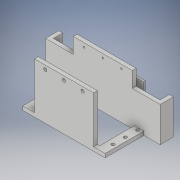
# Autodesk Inventor part: Frame
Saved by Autodesk Inventor 2019 (Build 230136000, 136)
## iProperties
Created: 2018-11-05
Part Number: Frame
Material: 일반
Document SubType Name: Modeling
Designer: otm09
Density: 1 g/cm^3
Appearance: 기본값
Author: otm09
Autodesk Inventor part; units mm, degrees
ref_plane "YZ Plane" through (0, 0, 0) normal (1, 0, 0) x (0, 1, 0)
ref_plane "XZ Plane" through (0, 0, 0) normal (0, 1, 0) x (-1, 0, 0)
ref_plane "XY Plane" through (0, 0, 0) normal (0, 0, 1) x (1, 0, 0)
sketch "스케치1" plane through (0, 0, 0) normal (0, 1, 0) x (-1, 0, 0)
  line L0 (0, 0) -> (106, 0)
  line L1 (106, 0) -> (106, -67)
  line L2 (106, -67) -> (0, -67)
  line L3 (0, -67) -> (0, 0)
  circle A0 centre (5, -15) radius 1.1
  circle A1 centre (5, -31) radius 1.1
  circle A2 centre (5, -47) radius 1.1
  circle A3 centre (101, -15) radius 1.1
  circle A4 centre (101, -31) radius 1.1
  circle A5 centre (101, -47) radius 1.1
  dimension "d1" = 2.2
  dimension "d4" = 16
  dimension "d7" = 96
  dimension "d10" = 5
  dimension "d11" = 15
  dimension "d12" = 5
  dimension "d13" = 20
  constraints: 8 end point, 6 centre point, 2 horizontal, 2 parallel, 1 perpendicular, 1 vertical, 10 other
  measures "d1" diameter of A0
  measures "d4" distance of A0.centre A1.centre
  measures "d7" distance of A0.centre A3.centre
  measures "d10" distance from line of L3 A0.centre
  measures "d11" distance from line of L0 A0.centre
  measures "d12" distance from line of L1 A3.centre
  measures "d13" distance from line of A2.centre L2
extrude "돌출1" add sketch "스케치1" along normal blind 5
sketch "스케치2" plane through (0, 5, 0) normal (0, 1, 0) x (1, 0, 0)
  circle A0 centre (-5, 15) radius 1.1 projected
  circle A1 centre (-5, 15) radius 2.1
  circle A2 centre (-5, 31) radius 1.1 projected
  circle A3 centre (-5, 31) radius 2.1
  circle A4 centre (-5, 47) radius 1.1 projected
  circle A5 centre (-5, 47) radius 2.1
  circle A6 centre (-101, 47) radius 1.1 projected
  circle A7 centre (-101, 47) radius 2.1
  circle A8 centre (-101, 31) radius 1.1 projected
  circle A9 centre (-101, 31) radius 2.1
  circle A10 centre (-101, 15) radius 1.1 projected
  circle A11 centre (-101, 15) radius 2.1
  point P0 (0, 0)
  dimension "d16" = 4.2
  dimension "d17" = 4.2
  dimension "d18" = 4.2
  dimension "d19" = 4.2
  dimension "d20" = 4.2
  dimension "d21" = 4.2
  constraints: 6 centre point, 6 coincident
  measures "d16" diameter of A1
  measures "d17" diameter of A3
  measures "d18" diameter of A5
  measures "d19" diameter of A7
  measures "d20" diameter of A9
  measures "d21" diameter of A11
extrude "돌출2" cut sketch "스케치2" against normal blind 3
sketch "스케치3" plane through (0, 5, 0) normal (0, 1, 0) x (1, 0, 0)
  line L0 (-106, 67) -> (0, 67) projected
  line L1 (-106, 0) -> (0, 0) projected
  line L2 (-91, 67) -> (-15, 67)
  line L3 (-15, 67) -> (-15, 0)
  line L4 (-15, 0) -> (-91, 0)
  line L5 (-91, 0) -> (-91, 67)
  line L6 (0, 0) -> (0, 67) projected
  line L7 (-106, 67) -> (-106, 0) projected
  line L8 (-91, 0) -> (-15, 0)
  line L9 (-15, 0) -> (-15, 5)
  line L10 (-15, 5) -> (-91, 5)
  line L11 (-91, 5) -> (-91, 0)
  line L12 (-91, 55) -> (-15, 55)
  line L13 (-15, 55) -> (-15, 50)
  line L14 (-15, 50) -> (-91, 50)
  line L15 (-91, 50) -> (-91, 55)
  dimension "d24" = 15
  dimension "d25" = 15
  dimension "d26" = 5
  dimension "d27" = 5
  dimension "d30" = 45
  constraints: 24 end point, 6 parallel, 6 point on line, 3 horizontal, 3 perpendicular, 1 collinear
  measures "d24" distance between parallel lines of L6 L3
  measures "d25" distance between parallel lines of L7 L5
  measures "d26" distance of L9.end L8.end
  measures "d27" distance of L12.end L13.end
  measures "d30" distance between parallel lines of L10 L14
extrude "돌출3" add sketch "스케치3" along normal blind 60 contours L12 L3 L14 L5 | L5 L10 L3 L1
sketch "스케치4" plane through (-106, 0, 0) normal (0, 0, 1) x (1, 0, 0)
  circle A0 centre (53, 60) radius 1.1
  circle A1 centre (77, 60) radius 1.1
  circle A2 centre (29, 60) radius 1.1
  line L0 (91, 5) -> (91, 65) projected
  line L1 (15, 65) -> (91, 65) projected
  point P0 (106, 0)
  dimension "d33" = 2.2
  dimension "d34" = 2.2
  dimension "d35" = 2.2
  dimension "d36" = 24
  dimension "d37" = 24
  dimension "d38" = 38
  dimension "d39" = 5
  dimension "d40" = 5
  dimension "d41" = 5
  constraints: 3 centre point
  measures "d33" diameter of A0
  measures "d34" diameter of A1
  measures "d35" diameter of A2
  measures "d36" distance of A2.centre A0.centre
  measures "d37" distance of A1.centre A0.centre
  measures "d38" distance from line of A0.centre L0
  measures "d39" distance from line of A0.centre L1
  measures "d40" distance from line of A1.centre L1
  measures "d41" distance from line of A2.centre L1
extrude "돌출4" cut sketch "스케치4" against normal blind 55
sketch "스케치5" plane through (-106, 0, 0) normal (0, 0, 1) x (1, 0, 0)
  circle A0 centre (29, 60) radius 1.1 projected
  circle A1 centre (29, 60) radius 2.1
  circle A2 centre (53, 60) radius 1.1 projected
  circle A3 centre (53, 60) radius 2.1
  circle A4 centre (77, 60) radius 1.1 projected
  circle A5 centre (77, 60) radius 2.1
  point P0 (106, 0)
  dimension "d44" = 4.2
  dimension "d45" = 4.2
  dimension "d46" = 4.2
  constraints: 3 centre point, 3 coincident
  measures "d44" diameter of A1
  measures "d45" diameter of A3
  measures "d46" diameter of A5
sketch "스케치6" plane through (-15, 5, -55) normal (0, 0, -1) x (-1, 0, 0)
  circle A0 centre (14, 55) radius 1.1 projected
  circle A1 centre (14, 55) radius 2.1
  circle A2 centre (38, 55) radius 1.1 projected
  circle A3 centre (38, 55) radius 2.1
  circle A4 centre (62, 55) radius 1.1 projected
  circle A5 centre (62, 55) radius 2.1
  point P0 (-15, -5)
  dimension "d47" = 4.2
  dimension "d48" = 4.2
  dimension "d49" = 4.2
  constraints: 3 centre point, 3 coincident
  measures "d47" diameter of A1
  measures "d48" diameter of A3
  measures "d49" diameter of A5
extrude "돌출5" cut sketch "스케치6" against normal blind 3
extrude "돌출6" cut sketch "스케치5" against normal blind 3
sketch "스케치7" plane through (0, 5, 0) normal (0, 1, 0) x (1, 0, 0)
  line L0 (-91, 67) -> (-15, 67)
  line L1 (-15, 67) -> (-15, 64.3)
  line L2 (-15, 64.3) -> (-91, 64.3)
  line L3 (-91, 64.3) -> (-91, 67)
  line L4 (-91, 55) -> (-91, 50) projected
  line L5 (-15, 50) -> (-15, 55) projected
  line L6 (-15, 55) -> (-91, 55) projected
  line L7 (-126.75, 50) -> (-121.75, 50)
  line L8 (-121.75, 50) -> (-121.75, 67)
  line L9 (-121.75, 67) -> (-126.75, 67)
  line L10 (-126.75, 67) -> (-126.75, 50)
  line L11 (15.75, 50) -> (20.75, 50)
  line L12 (20.75, 50) -> (20.75, 67)
  line L13 (20.75, 67) -> (15.75, 67)
  line L14 (15.75, 67) -> (15.75, 50)
  line L15 (-106, 67) -> (-106, 0) projected
  line L16 (-126.75, 50) -> (-106, 50)
  line L17 (-106, 50) -> (-106, 67)
  line L18 (-106, 67) -> (-126.75, 67)
  line L19 (-126.75, 67) -> (-126.75, 50)
  line L20 (0, 50) -> (20.75, 50)
  line L21 (20.75, 50) -> (20.75, 67)
  line L22 (20.75, 67) -> (0, 67)
  line L23 (0, 67) -> (0, 50)
  point P0 (0, 0)
  point P1 (0, 67)
  dimension "d54" = 9.3
  dimension "d56" = 5
  dimension "d57" = 5
  dimension "d58" = 137.5
  dimension "d59" = 15.75
  constraints: 40 end point, 10 parallel, 5 horizontal, 5 perpendicular, 3 point on line, 2 collinear
  measures "d54" distance between parallel lines of L2 L6
  measures "d56" distance of L9.end L8.end
  measures "d57" distance of L13.end L12.end
  measures "d58" distance between parallel lines of L14 L8
  measures "d59" distance between parallel lines of L15 L8
extrude "돌출7" add sketch "스케치7" along normal blind 40 contours L10 L9 L8 L7 | L14 L13 L12 L11
extrude "돌출8" add sketch "스케치7" against normal blind 5 contours L10 L9 L8 L7 | L8 L18 L15 L16 | L14 L13 L12 L11 | L20 L23 L22 L14
extrude "돌출9" add sketch "스케치7" along normal blind 40 contours L0 L1 L2 L3
sketch "스케치8" plane through (15.75, 5, -67) normal (-1, 0, 0) x (0, 0, 1)
  line L0 (17, 0) -> (12, 0) projected
  line L1 (17, 0) -> (12, 0)
  line L2 (12, 0) -> (12, 40)
  line L3 (12, 40) -> (17, 40)
  line L4 (17, 40) -> (17, 0)
  point P0 (67, -5)
  dimension "d66" = 5
  dimension "d67" = 40
  constraints: 8 end point, 2 parallel, 1 horizontal, 1 perpendicular
  measures "d66" distance of L2.end L3.end
  measures "d67" distance of L1.end L2.end
extrude "돌출10" add sketch "스케치8" along normal blind 142.5
sketch "스케치9" plane through (0, 5, 0) normal (0, 1, 0) x (1, 0, 0)
  line L0 (0, 50) -> (-106, 50) projected
  line L1 (-94, 5) -> (-12, 5)
  line L2 (-12, 5) -> (-12, 50)
  line L3 (-12, 50) -> (-94, 50)
  line L4 (-94, 50) -> (-94, 5)
  line L5 (-15, 5) -> (-91, 5) projected
  line L6 (-106, 50) -> (-106, 0) projected
  line L7 (0, 0) -> (0, 50) projected
  dimension "d70" = 12
  dimension "d71" = 12
  constraints: 8 end point, 2 parallel, 1 collinear, 1 horizontal, 1 perpendicular, 1 point on line
  measures "d70" distance between parallel lines of L4 L6
  measures "d71" distance between parallel lines of L7 L2
extrude "돌출11" cut sketch "스케치9" against normal blind 10
equation "\"d25\" = d24"
